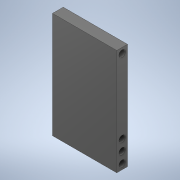
# Autodesk Inventor part: Part13
Saved by Autodesk Inventor 2020 (Build 240168000, 168)
## iProperties
Created: 2021-06-08
Part Number: Part13
Material: アセタール樹脂、黒
Document SubType Name: Modeling
Designer: masato
Density: 1.425 g/cm^3
Appearance: 滑らか - 黒
Author: masato
Autodesk Inventor part; units mm, degrees
ref_plane "YZ Plane" through (0, 0, 0) normal (1, 0, 0) x (0, 1, 0)
ref_plane "XZ Plane" through (0, 0, 0) normal (0, 1, 0) x (-1, 0, 0)
ref_plane "XY Plane" through (0, 0, 0) normal (0, 0, 1) x (1, 0, 0)
sketch "スケッチ1" plane through (0, 0, 0) normal (0, 0, 1) x (1, 0, 0)
  line L0 (0, 49.5) -> (30, 49.5)
  line L1 (0, 0) -> (30, 0)
  line L2 (0, 0) -> (0, 49.5)
  line L3 (30, 0) -> (30, 49.5)
  dimension "d2" = 30
  dimension "d38" = 49.5
  constraints: 8 end point, 2 parallel, 1 coincident, 1 perpendicular, 1 vertical
  measures "d2" distance of L0.start L0.end
  measures "d38" distance of L1.start L0.start
extrude "押し出し1" add sketch "スケッチ1" along normal blind 5
sketch "スケッチ4" plane through (30, 0, 0) normal (1, 0, 0) x (0, 0, -1)
  line L0 (0, 49.5) -> (-5, 49.5) projected
  line L1 (-2.5, 49.5) -> (-2.5, 0) construction
  line L2 (0, 0) -> (-5, 0) projected
  point P0 (0, 0)
  point P1 (-2.5, 47)
  point P2 (-2.5, 2.5)
  point P3 (-2.5, 7.5)
  point P4 (-2.5, 12.5)
  dimension "d22" = 2.5
  dimension "d40" = 2.5
  dimension "d41" = 5
  dimension "d42" = 5
  constraints: 4 point on line, 2 end point, 2 midpoint
  measures "d22" distance of L1.start point (-2.5, 47)
  measures "d40" distance of L1.end point (-2.5, 2.5)
  measures "d41" distance of point (-2.5, 2.5) point (-2.5, 7.5)
  measures "d42" distance of point (-2.5, 7.5) point (-2.5, 12.5)
hole "穴1" at (30, 47, 2.5) direction (-1, 0, 0) diameter 3.1 depth 5
sketch "スケッチ5" plane through (0, 0, 0) normal (-1, 0, 0) x (0, 0, 1)
  circle A0 centre (2.5, 47) radius 1.55 projected
  line L0 (0, 0) -> (5, 0) projected
  line L1 (2.5, 0) -> (2.5, 49.5) construction
  line L2 (0, 49.5) -> (5, 49.5) projected
  point P0 (2.5, 2.5)
  point P1 (2.5, 7.5)
  point P2 (2.5, 12.5)
  dimension "d50" = 2.5
  dimension "d51" = 5
  dimension "d52" = 5
  constraints: 3 point on line, 2 end point, 2 midpoint, 1 coincident
  measures "d50" distance of point (2.5, 2.5) L1.start
  measures "d51" distance of point (2.5, 7.5) point (2.5, 2.5)
  measures "d52" distance of point (2.5, 12.5) point (2.5, 7.5)
hole "穴2" at (0, 47, 2.5) direction (1, 0, 0) diameter 3.1 depth 5
hole "穴5" at (30, 2.5, 2.5) at (30, 12.5, 2.5) at (30, 7.5, 2.5) direction (-1, 0, 0) diameter 3 depth 3
hole "穴6" at (0, 2.5, 2.5) at (0, 7.5, 2.5) at (0, 12.5, 2.5) direction (1, 0, 0) diameter 3 depth 3
equation "\"d41\" = d42"
equation "\"d50\" = d40"
equation "\"d51\" = d41"
equation "\"d52\" = d42"
